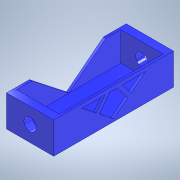
# Autodesk Inventor part: Motor Mount
Saved by Autodesk Inventor 2022 (Build 260153000, 153)
## iProperties
Created: 2022-08-10
Part Number: Motor Mount
Material: Generic
Document SubType Name: Modeling
Designer: Nick
Density: 1 g/cm^3
Appearance: Blue - Wall Paint - Glossy
Mass: 37.6373 g
Surface Area: 174.474 cm^2
Volume: 37.6373 cm^3
Author: Nick
Autodesk Inventor part; units mm, degrees
ref_plane "YZ Plane" through (0, 0, 0) normal (1, 0, 0) x (0, 1, 0)
ref_plane "XZ Plane" through (0, 0, 0) normal (0, 1, 0) x (-1, 0, 0)
ref_plane "XY Plane" through (0, 0, 0) normal (0, 0, 1) x (1, 0, 0)
sketch "Sketch14" plane through (0, 0, 0) normal (0, 0, 1) x (1, 0, 0)
  line L0 (0, 0) -> (60, 0)
  line L1 (60, 0) -> (60, 40)
  line L2 (60, 40) -> (0, 40)
  line L3 (0, 40) -> (0, 0)
  circle A0 centre (30, 20) radius 8
  point P0 (60, 20)
  point P1 (30, 40)
  dimension "d94" = 16
  dimension "d95" = 60
  dimension "d96" = 40
  constraints: 8 end point, 2 midpoint, 2 parallel, 1 centre point, 1 horizontal, 1 horizontal alignment, 1 perpendicular, 1 vertical alignment
  measures "d94" diameter of A0
  measures "d95" distance of L0.start L0.end
  measures "d96" distance of L2.end L0.start
extrude "Extrusion13" add sketch "Sketch14" along normal blind 10
sketch "Sketch15" plane through (0, 0, 0) normal (0, -1, 0) x (1, 0, 0)
  line L0 (0, 0) -> (60, 0) projected
  line L1 (60, 0) -> (60, 10) projected
  line L2 (0, 10) -> (60, 10) projected
  line L3 (0, 0) -> (0, 10) projected
  line L4 (60, 0) -> (60, 10) projected
  line L5 (60, 10) -> (0, 10)
  line L6 (0, 10) -> (0, 76.2)
  line L7 (0, 76.2) -> (60, 76.2)
  line L8 (60, 76.2) -> (60, 10)
  line L9 (0, 0) -> (0, 10) projected
  dimension "d99" = 66.2
  constraints: 8 end point, 2 parallel, 1 collinear, 1 horizontal, 1 perpendicular
  measures "d99" distance of L7.end L1.end
extrude "Extrusion14" add sketch "Sketch15" against normal blind 3 contours L6 L7 L8 L2
sketch "Sketch16" plane through (60, 0, 0) normal (1, 0, 0) x (0, 0, -1)
  line L0 (0, 0) -> (0, 40) projected
  line L1 (0, 40) -> (-10, 40) projected
  line L2 (-10, 3) -> (-10, 40) projected
  line L3 (-76.2, 3) -> (-10, 3) projected
  line L4 (-76.2, 0) -> (-76.2, 3) projected
  line L5 (0, 0) -> (-76.2, 0) projected
  line L6 (0, 40) -> (-10, 40) projected
  line L7 (-10, 3) -> (-76.2, 3) projected
  line L8 (-10, 3) -> (-10, 40) projected
  line L9 (-10, 40) -> (-29.0932, 40)
  line L10 (-29.0932, 40) -> (-76.2, 3)
  point P0 (0, 0)
  dimension "d106" = 29.0932
  constraints: 4 end point, 1 horizontal
  measures "d106" distance from line of L0 L9.end
extrude "Extrusion15" add sketch "Sketch16" against normal blind 3 contours L2 L3 L10 L9
ref_plane "Work Plane3" through (30, 0, 0) normal (1, 0, 0) x (0, 0, -1)
mirror "Mirror3" about plane through (30, 0, 0) normal (1, 0, 0) of "Extrusion15"
mirror "Mirror4" about plane through (0, 0, 76.2) normal (0, 0, 1)
sketch "Sketch17" plane through (60, 0, 0) normal (1, 0, 0) x (0, 0, -1)
  line L0 (0, 0) -> (0, 40) projected
  line L1 (0, 40) -> (-29.0932, 40) projected
  line L2 (-29.0932, 40) -> (-76.2, 3) projected
  line L3 (-123.3068, 40) -> (-76.2, 3) projected
  line L4 (-152.4, 40) -> (-123.3068, 40) projected
  line L5 (-152.4, 0) -> (-152.4, 40) projected
  line L6 (-152.4, 0) -> (0, 0) projected
  line L7 (-152.4, 40) -> (-123.3068, 40) projected
  line L8 (-76.2, 3) -> (-29.0932, 40) projected
  line L9 (-123.3068, 40) -> (-29.0932, 40)
  line L10 (-76.2, 3) -> (-123.3068, 40) projected
  line L11 (-116.9411, 35) -> (-35.4589, 35)
  line L12 (-98.5366, 20.5442) -> (-87.1823, 35)
  line L13 (-65.2177, 35) -> (-53.8634, 20.5442)
  line L14 (-29.0932, 40) -> (-76.2, 3) projected
  line L15 (-123.3068, 40) -> (-76.2, 3) projected
  line L16 (-94.6045, 17.4558) -> (-80.8244, 35)
  line L17 (-71.5756, 35) -> (-57.7955, 17.4558)
  line L18 (-57.7955, 17.4558) -> (-53.8634, 20.5442)
  line L19 (-76.2, 3) -> (-35.4589, 35)
  line L20 (-116.9411, 35) -> (-76.2, 3)
  line L21 (-98.5366, 20.5442) -> (-94.6045, 17.4558)
  point P0 (0, 0)
  point P1 (-55.8295, 19)
  point P2 (-96.5705, 19)
  dimension "d107" = 5
  dimension "d110" = 5
  dimension "d111" = 5
  constraints: 20 end point, 10 point on line, 4 midpoint, 4 perpendicular, 3 collinear, 2 horizontal
  measures "d107" distance between parallel lines of L9 L11
  measures "d110" distance between parallel lines of L16 L12
  measures "d111" distance between parallel lines of L13 L17
extrude "Extrusion16" add sketch "Sketch17" against normal blind 3 contours L2 L11 L3 L9 | L2 L17 L11 L13 | L12 L11 L16 L3
body "Solid3"
